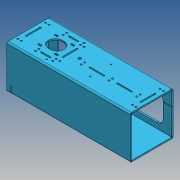
# Autodesk Inventor part: Case2
Saved by Autodesk Inventor 2017 (Build 210142000, 142)
## iProperties
Part Number: Case2
Material: Genérico
Document SubType Name: Chapa
Designer: Leo
Density: 1 g/cm^3
Appearance: Turquesa
Sheet Metal Rule: Por defecto
Flat Pattern Width: 51.442 cm
Flat Pattern Length: 35.5 cm
Flat Pattern Area: 1826.19 cm^2
Sheet Metal Width: 514,420 mm
Sheet Metal Length: 355,000 mm
Sheet Metal Area: 182619,121 mm^2
Author: Leo
Autodesk Inventor part; units mm, degrees
ref_plane "YZ Plane" through (0, 0, 0) normal (1, 0, 0) x (0, 1, 0)
ref_plane "XZ Plane" through (0, 0, 0) normal (0, 1, 0) x (-1, 0, 0)
ref_plane "XY Plane" through (0, 0, 0) normal (0, 0, 1) x (1, 0, 0)
sketch "Boceto1" plane through (0, 0, 0) normal (0, 0, 1) x (1, 0, 0)
  circle A0 centre (0, 0) radius 4.805 construction
  circle A1 centre (0, 0) radius 10 construction
  circle A2 centre (67.5, 0) radius 57.5 construction
  line L0 (28.2, 28.2) -> (-28.2, 28.2) construction
  line L1 (-28.2, 28.2) -> (-28.2, -28.2) construction
  line L2 (-28.2, -28.2) -> (28.2, -28.2) construction
  line L3 (28.2, -28.2) -> (28.2, 28.2) construction
  line L4 (-7.037, 7.1049) -> (27.037, 40.8534) construction
  line L5 (27.037, -40.8534) -> (-7.037, -7.1049) construction
  line L6 (51.8, -14) -> (251.8, -14) construction
  line L7 (251.8, -14) -> (251.8, -56) construction
  line L8 (251.8, -56) -> (51.8, -56) construction
  line L9 (51.8, -56) -> (51.8, -14) construction
  circle A3 centre (67.5, 0) radius 4
  line L10 (-20.57, 21.07) -> (-26.57, 21.07)
  arc A4 (-26.57, 26.07) -> (-26.57, 21.07) centre (-26.57, 23.57) ccw
  line L11 (-26.57, 26.07) -> (-20.57, 26.07)
  arc A5 (-20.57, 21.07) -> (-20.57, 26.07) centre (-20.57, 23.57) ccw
  line L12 (20.57, -21.07) -> (26.57, -21.07)
  arc A6 (26.57, -26.07) -> (26.57, -21.07) centre (26.57, -23.57) ccw
  line L13 (26.57, -26.07) -> (20.57, -26.07)
  arc A7 (20.57, -21.07) -> (20.57, -26.07) centre (20.57, -23.57) ccw
  line L14 (20.57, 26.07) -> (26.57, 26.07)
  arc A8 (26.57, 21.07) -> (26.57, 26.07) centre (26.57, 23.57) ccw
  line L15 (26.57, 21.07) -> (20.57, 21.07)
  arc A9 (20.57, 26.07) -> (20.57, 21.07) centre (20.57, 23.57) ccw
  line L16 (-20.57, 23.57) -> (-26.57, 23.57) construction
  line L17 (20.57, 23.57) -> (26.57, 23.57) construction
  line L18 (48.6318, 0) -> (86.3682, 0) construction
  circle A10 centre (127.9669, 30) radius 2
  circle A11 centre (127.9669, -30) radius 2
  circle A12 centre (127.9669, 30) radius 10 construction
  circle A13 centre (67.5, 0) radius 30 construction
  line L19 (126.2385, 20.1505) -> (72.6854, 29.5485) construction
  line L20 (-78.2, 60) -> (276.8, 60)
  line L21 (276.8, 60) -> (276.8, -60)
  line L22 (276.8, -60) -> (-78.2, -60)
  line L23 (-78.2, -60) -> (-78.2, 60)
  circle A14 centre (22.1541, -50) radius 2
  circle A15 centre (22.1541, -50) radius 10 construction
  circle A16 centre (67.5, 0) radius 11 construction
  line L24 (-26.57, -21.07) -> (-20.57, -21.07)
  arc A17 (-20.57, -26.07) -> (-20.57, -21.07) centre (-20.57, -23.57) ccw
  line L25 (-20.57, -26.07) -> (-26.57, -26.07)
  arc A18 (-26.57, -21.07) -> (-26.57, -26.07) centre (-26.57, -23.57) ccw
  line L26 (-26.57, -23.57) -> (-20.57, -23.57) construction
  line L27 (-23.57, -23.57) -> (-23.57, 23.57) construction
  line L28 (23.57, 23.57) -> (23.57, -18.9602) construction
  line L29 (-23.57, 0) -> (23.57, 0) construction
  line L30 (-3, -20) -> (3, -20)
  arc A19 (3, -20) -> (3, 20) centre (3, 0) ccw
  line L31 (3, 20) -> (-3, 20)
  arc A20 (-3, 20) -> (-3, -20) centre (-3, 0) ccw
  line L32 (-67.7, 20.5) -> (-67.7, -20.5)
  arc A21 (-67.7, -20.5) -> (-63.7, -20.5) centre (-65.7, -20.5) ccw
  line L33 (-63.7, -20.5) -> (-63.7, 20.5)
  arc A22 (-63.7, 20.5) -> (-67.7, 20.5) centre (-65.7, 20.5) ccw
  circle A23 centre (-70.7, -40) radius 2.5
  circle A24 centre (-60.7, -40) radius 2.5
  line L34 (-70.7, -40) -> (-60.7, -40) construction
  circle A25 centre (-70.7, 40) radius 2.5
  circle A26 centre (-60.7, 40) radius 2.5
  line L35 (266.3, 20.5) -> (266.3, -20.5)
  arc A27 (262.3, -20.5) -> (266.3, -20.5) centre (264.3, -20.5) ccw
  line L36 (262.3, -20.5) -> (262.3, 20.5)
  arc A28 (266.3, 20.5) -> (262.3, 20.5) centre (264.3, 20.5) ccw
  line L37 (99.3, 60) -> (99.3, -60) construction
  circle A29 centre (269.3, -40) radius 2.5
  circle A30 centre (259.3, -40) radius 2.5
  circle A31 centre (259.3, 40) radius 2.5
  circle A32 centre (269.3, 40) radius 2.5
  line L38 (38, 20.5) -> (38, -20.5)
  arc A33 (38, -20.5) -> (42, -20.5) centre (40, -20.5) ccw
  line L39 (42, -20.5) -> (42, 20.5)
  arc A34 (42, 20.5) -> (38, 20.5) centre (40, 20.5) ccw
  line L40 (-3, 38) -> (23, 38)
  arc A35 (23, 38) -> (23, 42) centre (23, 40) ccw
  line L41 (23, 42) -> (-3, 42)
  arc A36 (-3, 42) -> (-3, 38) centre (-3, 40) ccw
  line L42 (-3, -38) -> (23, -38)
  arc A37 (23, -42) -> (23, -38) centre (23, -40) ccw
  line L43 (23, -42) -> (-3, -42)
  arc A38 (-3, -38) -> (-3, -42) centre (-3, -40) ccw
  line L44 (104.4, -10) -> (145.4, -10)
  arc A39 (145.4, -10) -> (145.4, -6) centre (145.4, -8) ccw
  line L45 (145.4, -6) -> (104.4, -6)
  arc A40 (104.4, -6) -> (104.4, -10) centre (104.4, -8) ccw
  line L46 (84.9, -3) -> (84.9, -13) construction
  circle A41 centre (84.9, -3) radius 2.5
  circle A42 centre (84.9, -13) radius 2.5
  line L47 (124.9, -10) -> (124.9, -6) construction
  circle A43 centre (164.9, -3) radius 2.5
  circle A44 centre (164.9, -13) radius 2.5
  line L48 (164.9, -13) -> (164.9, -3) construction
  line L49 (225.4, -10) -> (184.4, -10)
  arc A45 (184.4, -6) -> (184.4, -10) centre (184.4, -8) ccw
  line L50 (184.4, -6) -> (225.4, -6)
  arc A46 (225.4, -10) -> (225.4, -6) centre (225.4, -8) ccw
  circle A47 centre (244.9, -3) radius 2.5
  circle A48 centre (244.9, -13) radius 2.5
  line L51 (10, -42) -> (10, -38) construction
  circle A49 centre (-15, -35) radius 2.5
  circle A50 centre (-15, -45) radius 2.5
  line L52 (-15, -45) -> (-15, -35) construction
  circle A51 centre (35, -35) radius 2.5
  circle A52 centre (35, -45) radius 2.5
  line L53 (42, 0) -> (38, 0) construction
  line L54 (35, -35) -> (45, -35) construction
  line L55 (40, -20.5) -> (40, 20.5) construction
  circle A53 centre (45, -35) radius 2.5
  circle A54 centre (-15, 35) radius 2.5
  circle A55 centre (-15, 45) radius 2.5
  circle A56 centre (35, 35) radius 2.5
  circle A57 centre (35, 45) radius 2.5
  circle A58 centre (45, 35) radius 2.5
  point P0 (-28.2, 0)
  point P1 (0, -28.2)
  point P2 (276.8, 0)
  point P3 (0, 20)
  point P4 (-67.7, 0)
  point P5 (-78.2, 0)
  point P6 (-65.7, -40)
  point P7 (84.9, -8)
  point P8 (-15, -40)
  point P9 (10, -40)
  point P10 (40, 0)
  point P11 (40, -35)
  dimension "d15" = 20
  dimension "d17" = 60
  dimension "d1" = 56.4
  dimension "d2" = 67.5
  dimension "d4" = 200
  dimension "d5" = 42
  dimension "d6" = 8
  dimension "d8" = 5
  dimension "d9" = 41.14
  dimension "d10" = 6
  dimension "d11" = 53.14
  dimension "d12" = 6
  dimension "d13" = 4
  dimension "d14" = 115
  dimension "d16" = 60
  dimension "d18" = 4
  dimension "d19" = 33.93
  dimension "d20" = 22
  dimension "d21" = 120
  dimension "d22" = 130
  dimension "d23" = 20
  dimension "d42" = 47.14
  dimension "d43" = 47.14
  dimension "d44" = 20
  dimension "d45" = 6
  dimension "d46" = 14.2
  dimension "d47" = 25
  dimension "d62" = 4
  dimension "d63" = 41
  dimension "d65" = 5
  dimension "d66" = 10
  dimension "d67" = 5
  dimension "d68" = 40
  dimension "d70" = 4
  dimension "d86" = 50
  dimension "d87" = 355
  dimension "d88" = 12.5
  dimension "d89" = 12.5
  dimension "d90" = 23.6
  dimension "d91" = 11.8
  dimension "d92" = 26
  dimension "d93" = 15
  dimension "d94" = 80
  dimension "d95" = 40
  dimension "d96" = 4
  dimension "d97" = 194.8
  dimension "d98" = 97.4
  constraints: 113 end point, 57 centre point, 52 point on circle, 47 tangent, 29 symmetric about line, 26 midpoint, 17 parallel, 13 horizontal, 13 horizontal alignment, 12 equal radius, 10 coincident, 8 vertical, 7 equal length, 7 vertical alignment, 5 perpendicular, 3 point on line, 1 collinear, 1 concentric, 33 other
  measures "d1" distance of L0.end L1.end
  measures "d2" distance of A2.centre point (0, 0)
  measures "d4" distance of L7.end L8.end
  measures "d5" distance of L6.end L7.end
  measures "d6" diameter of A3
  measures "d8" distance between parallel lines of L11 L10
  measures "d9" distance of L17.start L16.start
  measures "d10" distance of L16.start L16.end
  measures "d11" distance of L17.end L16.end
  measures "d12" distance of L16.start L16.end
  measures "d13" diameter of A10
  measures "d14" diameter of A2
  measures "d16" distance of point (127.967, 30) A11.centre
  measures "d18" distance between parallel lines of L22 L8
  measures "d19" distance edge to line of A4 L20
  measures "d20" diameter of A16
  measures "d21" distance of L20.end L21.end
  measures "d22" distance between parallel lines of L23 L9
  measures "d23" diameter of A15
  measures "d42" distance from line of L26.start L16
  measures "d43" distance between parallel lines of L28 L27
  measures "d44" radius of A20
  measures "d45" distance of L30.start L30.end
  measures "d46" distance between parallel lines of L2 L6
  measures "d47" distance between parallel lines of L21 L7
  measures "d62" distance between parallel lines of L33 L32
  measures "d63" distance of L32.start L32.end
  measures "d65" diameter of A24
  measures "d66" distance of L34.start L34.end
  measures "d67" distance edge to line of A23 L23
  measures "d68" distance from line of L34 point (-67.7, 0)
  measures "d70" distance between parallel lines of L36 L35
  measures "d86" distance between parallel lines of L23 L1
  measures "d87" distance of L20.start L20.end
  measures "d88" distance from line of A22.centre L23
  measures "d89" distance from line of A28.centre L21
  measures "d90" distance between parallel lines of L3 L9
  measures "d91" distance from line of L55.start L3
  measures "d92" distance of L41.start L41.end
  measures "d93" distance from line of A35.centre L38
  measures "d94" distance of A38.centre A36.centre
  measures "d95" distance between parallel lines of L46 L47
  measures "d96" distance between parallel lines of L49 L6
  measures "d97" distance from line of L36 A2.centre
  measures "d98" distance between parallel lines of L48 L36
extrude "Extrusión1" add sketch "Boceto1" along normal blind 4
sketch "Boceto3" plane through (-68.7083, 50.17, -120) normal (0, 1, 0) x (1, 0, 0)
  line L0 (0, -119.9) -> (265, -119.9) construction
  line L1 (265, 0) -> (265, -119.9) construction
  line L2 (0, 0) -> (265, 0) construction
  line L3 (0, -119.9) -> (0, 0) construction
  line L4 (136.5, -57.95) -> (128.5, -57.95)
  arc A0 (128.5, -57.95) -> (128.5, -61.95) centre (128.5, -59.95) ccw
  line L5 (128.5, -61.95) -> (136.5, -61.95)
  arc A1 (136.5, -61.95) -> (136.5, -57.95) centre (136.5, -59.95) ccw
  line L6 (238, -57.95) -> (230, -57.95)
  arc A2 (230, -57.95) -> (230, -61.95) centre (230, -59.95) ccw
  line L7 (230, -61.95) -> (238, -61.95)
  arc A3 (238, -61.95) -> (238, -57.95) centre (238, -59.95) ccw
  line L8 (35, -57.95) -> (27, -57.95)
  arc A4 (27, -57.95) -> (27, -61.95) centre (27, -59.95) ccw
  line L9 (27, -61.95) -> (35, -61.95)
  arc A5 (35, -61.95) -> (35, -57.95) centre (35, -59.95) ccw
  point P0 (68.7083, -120)
  point P1 (265, -59.95)
  point P2 (132.5, 0)
  point P3 (132.5, -57.95)
  dimension "d36" = 4
  dimension "d37" = 8
  dimension "d38" = 25
  dimension "d39" = 25
  constraints: 12 end point, 12 point on circle, 12 tangent, 6 centre point, 3 horizontal, 3 horizontal alignment, 3 midpoint, 3 parallel, 2 collinear, 2 equal radius, 1 vertical alignment
  measures "d36" distance between parallel lines of L5 L4
  measures "d37" distance of L5.start L5.end
  measures "d38" distance edge to line of A4 L3
  measures "d39" distance edge to line of A3 L1
sketch "Boceto2" plane through (-78.2, -60.1, -0.1) normal (0, -1, 0) x (1, 0, 0)
  line L0 (355, 0) -> (0, 0)
  line L1 (0, 0) -> (0, -119.9)
  line L2 (0, -119.9) -> (355, -119.9)
  line L3 (355, -119.9) -> (355, 0)
  constraints: 6 end point, 1 horizontal, 1 perpendicular, 1 vertical
edge flange "Pestaña1" height 120 angle 90 thickness 4 bend radius 0.1 thickness toward (0, -1, 0) relief tear relief width 4 relief depth 2 edges at (99.3, -60, 0) wall of the first edge with corners at (276.8, -60.1, -0.1) (-78.2, -60.1, -0.1) (-78.2, -60.1, -120) (276.8, -60.1, -120)
bend "Doblez1"
corner "Esquina1"
sketch "Boceto4" plane through (-78.2, 60, 0) normal (0, 1, 0) x (1, 0, 0)
  line L0 (355, 120) -> (0, 120)
  line L1 (0, 0) -> (355, 0)
  line L2 (0, 120) -> (0, 80.1667)
  line L3 (0, 80.1667) -> (25, 80.1667)
  line L4 (25, 80.1667) -> (25, 83.4303)
  arc A0 (41.5697, 100) -> (25, 83.4303) centre (41.5697, 83.4303) ccw
  line L5 (41.5697, 100) -> (313.4303, 100)
  arc A1 (330, 83.4303) -> (313.4303, 100) centre (313.4303, 83.4303) ccw
  line L6 (330, 83.4303) -> (330, 40.3333)
  line L7 (330, 40.3333) -> (355, 40.3333)
  line L8 (355, 120) -> (355, 40.3333)
  line L9 (355, 0) -> (355, 39.8333)
  line L10 (355, 39.8333) -> (330, 39.8333)
  line L11 (330, 39.8333) -> (330, 36.5697)
  arc A2 (313.4303, 20) -> (330, 36.5697) centre (313.4303, 36.5697) ccw
  line L12 (313.4303, 20) -> (41.5697, 20)
  arc A3 (25, 36.5697) -> (41.5697, 20) centre (41.5697, 36.5697) ccw
  line L13 (25, 36.5697) -> (25, 79.6667)
  line L14 (25, 79.6667) -> (0, 79.6667)
  line L15 (0, 79.6667) -> (0, 0)
  line L16 (344.5, 27.7391) -> (344.5, 68.7391)
  arc A4 (344.5, 68.7391) -> (340.5, 68.7391) centre (342.5, 68.7391) ccw
  line L17 (340.5, 68.7391) -> (340.5, 27.7391)
  arc A5 (340.5, 27.7391) -> (344.5, 27.7391) centre (342.5, 27.7391) ccw
  line L18 (10.5, 51.123) -> (10.5, 92.123)
  arc A6 (14.5, 92.123) -> (10.5, 92.123) centre (12.5, 92.123) ccw
  line L19 (14.5, 92.123) -> (14.5, 51.123)
  arc A7 (10.5, 51.123) -> (14.5, 51.123) centre (12.5, 51.123) ccw
  point P0 (196.907, 99.9603)
  point P1 (0, 120)
  point P2 (342.5, 39.8333)
  point P3 (12.5, 79.6667)
  dimension "d58" = 0.5
  dimension "d59" = 0.5
  dimension "d60" = 20
  dimension "d61" = 20
  dimension "d71" = 25
  dimension "d72" = 25
  dimension "d78" = 4
  dimension "d79" = 41
  dimension "d80" = 39.8333
  dimension "d81" = 79.6667
  constraints: 40 end point, 16 point on circle, 16 tangent, 10 perpendicular, 8 centre point, 6 vertical, 4 coincident, 4 equal radius, 4 parallel, 2 collinear, 2 midpoint, 2 vertical alignment
  measures "d58" distance between parallel lines of L10 L7
  measures "d59" distance between parallel lines of L14 L3
  measures "d60" distance between parallel lines of L1 L12
  measures "d61" distance between parallel lines of L0 L5
  measures "d71" distance between parallel lines of L15 L13
  measures "d72" distance between parallel lines of L8 L6
  measures "d78" distance between parallel lines of L17 L16
  measures "d79" distance of L16.start L16.end
  measures "d80" distance of L1.end L9.end
  measures "d81" distance of L0.start L7.end
sheet face with bend "Cara1" sketch "Boceto4" thickness 4 toward (0, -1, 0) bend radius 0.1 relief tear relief width 4 relief depth 2 contours L8 L7 L16 A4 L17 L6 A1 L5 A0 L4 L3 L19 A6 L18 L2 L0 | L7 L17 A4 L16 | L18 A6 L19 L3
bend "Doblez2"
sheet face with bend "Cara2" sketch "Boceto4" thickness 4 toward (0, -1, 0) bend radius 0.1 relief tear relief width 4 relief depth 2 contours L16 A5 L17 L10 | L10 L9 L1 L15 L14 L18 A7 L19 L13 A3 L12 A2 L11 L17 A5 L16 | L14 L19 A7 L18
bend "Doblez3"
sketch "Boceto5" plane through (276.8, 60, -120) normal (0, 0, -1) x (-1, 0, 0)
  line L0 (0, -4) -> (355, -4) projected
  line L1 (0, -120.1) -> (355, -120.1) projected
  line L2 (355, 0) -> (355, -4) projected
  line L3 (355, -4) -> (355, -120.1)
  line L4 (0, -120.1) -> (0, -4)
  line L5 (344.5, -80.5) -> (344.5, -39.5) projected
  arc A0 (344.5, -39.5) -> (340.5, -39.5) centre (342.5, -39.5) ccw projected
  line L6 (340.5, -39.5) -> (340.5, -80.5) projected
  arc A1 (340.5, -80.5) -> (344.5, -80.5) centre (342.5, -80.5) ccw projected
  line L7 (344.5, 1) -> (344.5, -20.05)
  arc A2 (340.5, -20.05) -> (344.5, -20.05) centre (342.5, -20.05) ccw
  line L8 (340.5, -20.05) -> (340.5, 1)
  line L9 (340.5, 1) -> (344.5, 1)
  line L10 (355, -4.1) -> (355, -120) projected
  line L11 (355, -62.05) -> (321.347, -62.05)
  line L12 (344.5, -125.1) -> (344.5, -104.05)
  arc A3 (344.5, -104.05) -> (340.5, -104.05) centre (342.5, -104.05) ccw
  line L13 (340.5, -104.05) -> (340.5, -125.1)
  line L14 (340.5, -125.1) -> (344.5, -125.1)
  point P0 (276.8, -60)
  dimension "d82" = 84
  dimension "d83" = 5
  constraints: 18 end point, 4 perpendicular, 4 point on circle, 4 tangent, 2 centre point, 2 collinear, 2 parallel, 2 vertical, 1 horizontal, 1 midpoint, 3 other
  measures "d82" distance of A3.centre A2.centre
  measures "d83" distance between parallel lines of L14 L1
sheet face with bend "Cara3" sketch "Boceto5" thickness 4 toward (0, 0, 1) bend radius 0.1 relief tear relief width 4 relief depth 2 contours L0 L8 A2 L7 L3 L1 L12 A3 L13 L4 | L0 L7 A2 L8 | L13 A3 L12 L1 | A1 L6 L11 L5 | L11 L6 A0 L5
bend "Doblez4"
extrude "Extrusión3" cut sketch "Boceto5" against normal blind 20 contours L8 L9 L7 L0 | L0 L7 A2 L8 | L13 A3 L12 L1 | L1 L12 L14 L13
